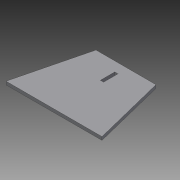
# Autodesk Inventor part: Side
Saved by Autodesk Inventor 2014 (Build 180170000, 170)
## iProperties
Created: 2015-02-09
Part Number: Side
Material: Generic
Document SubType Name: Modeling
Designer: ThatOtherGuy
Density: 1 g/cm^3
Appearance: Default
Author: ThatOtherGuy
Autodesk Inventor part; units mm, degrees
ref_plane "YZ Plane" through (0, 0, 0) normal (1, 0, 0) x (0, 1, 0)
ref_plane "XZ Plane" through (0, 0, 0) normal (0, 1, 0) x (-1, 0, 0)
ref_plane "XY Plane" through (0, 0, 0) normal (0, 0, 1) x (1, 0, 0)
sketch "Sketch1" plane through (0, 0, 0) normal (0, 0, 1) x (1, 0, 0)
  line L0 (0, 0) -> (200, 0)
  line L1 (200, 0) -> (162.5, 150)
  line L2 (162.5, 150) -> (37.5, 150)
  line L3 (37.5, 150) -> (0, 0)
  dimension "d0" = 150
  dimension "d1" = 200
  dimension "d2" = 125
  constraints: 8 end point, 1 equal length, 1 horizontal, 1 parallel
  measures "d0" distance between parallel lines of L0 L2
  measures "d1" distance of L0.start L0.end
  measures "d2" distance of L1.end L2.end
extrude "Extrusion1" add sketch "Sketch1" along normal blind 6.731
sketch "Sketch2" plane through (0, 0, 6.731) normal (0, 0, 1) x (1, 0, 0)
  line L0 (0, 0) -> (200, 0) projected
  line L1 (162.5, 150) -> (37.5, 150) projected
  line L2 (96.6345, 130) -> (103.3655, 130)
  line L3 (103.3655, 130) -> (103.3655, 100)
  line L4 (103.3655, 100) -> (96.6345, 100)
  line L5 (96.6345, 100) -> (96.6345, 130)
  point P0 (100, 130)
  point P1 (100, 150)
  dimension "d5" = 30
  dimension "d6" = 100
  dimension "d7" = 6.731
  constraints: 8 end point, 2 midpoint, 2 parallel, 1 horizontal, 1 perpendicular, 1 vertical alignment
  measures "d5" distance of L2.end L3.end
  measures "d6" distance between parallel lines of L0 L4
  measures "d7" distance of L2.start L2.end
extrude "Extrusion2" cut sketch "Sketch2" against normal up to next
equation "\"d3\" = THICKB"
equation "\"d7\" = THICKB"
equation "\"THICKA\" = 3.175"
equation "\"THICKB\" = 6.731"
equation "\"THICKC\" = 12.7"
equation "\"THICKPLY\" = 5"
equation "\"MAGDIA\" = 9.5"
equation "\"BALLDIA\" = 12"
body "Solid1"
